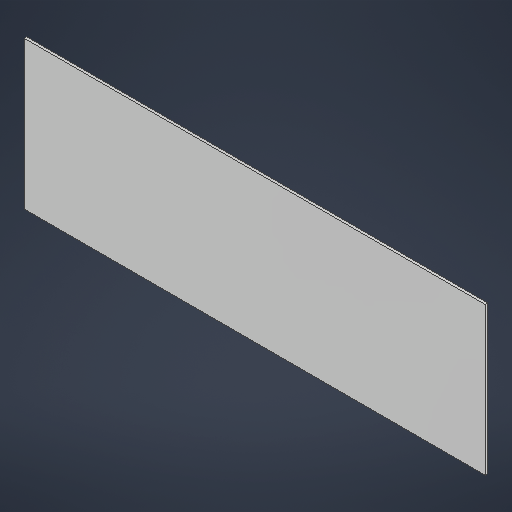
# Autodesk Inventor part: Mecanismo_base_al
Saved by Autodesk Inventor 2026 (Build 300175050, 175E)
## iProperties
Created: 2025-11-11
Part Number: Mecanismo_base_al
Material: Generic
Document SubType Name: Modeling
Designer: habbo
Density: 1 g/cm^3
Appearance: Aluminum - Polished
Author: habbo
Autodesk Inventor part; units mm, degrees
ref_plane "YZ Plane" through (0, 0, 0) normal (1, 0, 0) x (0, 1, 0)
ref_plane "XZ Plane" through (0, 0, 0) normal (0, 1, 0) x (-1, 0, 0)
ref_plane "XY Plane" through (0, 0, 0) normal (0, 0, 1) x (1, 0, 0)
sketch "Sketch1" plane through (0, 0, 0) normal (0, 0, 1) x (1, 0, 0)
  line L0 (-265, -85) -> (265, -85)
  line L1 (265, -85) -> (265, 85)
  line L2 (265, 85) -> (-265, 85)
  line L3 (-265, 85) -> (-265, -85)
  line L4 (-265, -85) -> (265, 85) construction
  line L5 (265, -85) -> (-265, 85) construction
  point P0 (0, 0)
  dimension "d0" = 530
  dimension "d1" = 170
  constraints: 12 end point, 2 midpoint, 2 parallel, 1 horizontal, 1 perpendicular
  measures "d0" distance of L2.end L1.end
  measures "d1" distance of L1.end L0.end
extrude "Extrusion1" add sketch "Sketch1" along normal mid plane 3
body "Solid1"
